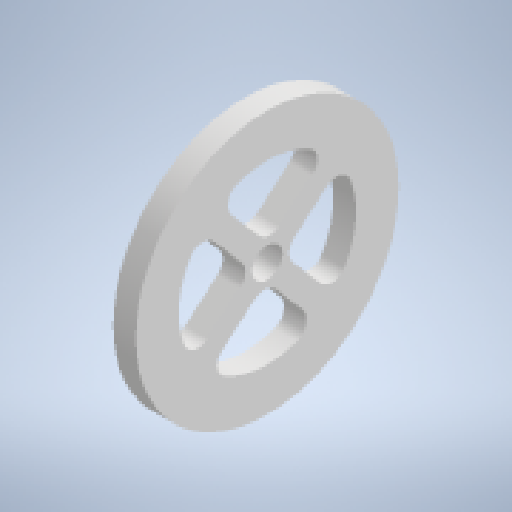
# Autodesk Inventor part: Wheel
Saved by Autodesk Inventor 2025.2 (Build 292293000, 293)
## iProperties
Created: 2025-02-03
Part Number: Wheel
Material: Generic
Document SubType Name: Modeling
Designer: andre
Density: 1 g/cm^3
Appearance: Default
Author: andre
Autodesk Inventor part; units mm, degrees
ref_plane "YZ Plane" through (0, 0, 0) normal (1, 0, 0) x (0, 1, 0)
ref_plane "XZ Plane" through (0, 0, 0) normal (0, 1, 0) x (-1, 0, 0)
ref_plane "XY Plane" through (0, 0, 0) normal (0, 0, 1) x (1, 0, 0)
sketch "Sketch1" plane through (0, 0, 0) normal (1, 0, 0) x (0, 1, 0)
  arc A0 (-4.9982, 77.0065) -> (-5.7361, 67.4907) centre (5.338, 71.4184) ccw
  arc A1 (-1.7195, 77.356) -> (-4.9982, 77.0065) centre (-3.2388, 76.0553) ccw
  line L0 (-1.7195, 77.356) -> (1.9224, 73.1018)
  arc A2 (1.7037, 70.2818) -> (1.9224, 73.1018) centre (0.4031, 71.8011) ccw
  line L1 (1.7037, 70.2818) -> (-2.5505, 66.6399)
  arc A3 (-5.7361, 67.4907) -> (-2.5505, 66.6399) centre (-3.8511, 68.1592) ccw
  arc A4 (-0.2501, 61.0823) -> (9.2657, 60.3443) centre (5.338, 71.4184) ccw
  arc A5 (-0.5995, 64.3609) -> (-0.2501, 61.0823) centre (0.7011, 62.8416) ccw
  line L2 (-0.5995, 64.3609) -> (3.6547, 68.0028)
  arc A6 (6.4746, 67.7841) -> (3.6547, 68.0028) centre (4.9553, 66.4835) ccw
  line L3 (6.4746, 67.7841) -> (10.1165, 63.5299)
  arc A7 (9.2657, 60.3443) -> (10.1165, 63.5299) centre (8.5972, 62.2293) ccw
  arc A8 (15.6742, 65.8304) -> (16.4121, 75.3462) centre (5.338, 71.4184) ccw
  arc A9 (12.3955, 65.4809) -> (15.6742, 65.8304) centre (13.9148, 66.7815) ccw
  line L4 (12.3955, 65.4809) -> (8.7536, 69.7351)
  arc A10 (8.9723, 72.5551) -> (8.7536, 69.7351) centre (10.2729, 71.0357) ccw
  line L5 (8.9723, 72.5551) -> (13.2265, 76.1969)
  arc A11 (16.4121, 75.3462) -> (13.2265, 76.1969) centre (14.5271, 74.6776) ccw
  line L6 (4.2014, 75.0527) -> (0.5595, 79.3069)
  arc A12 (1.4103, 82.4925) -> (0.5595, 79.3069) centre (2.0788, 80.6076) ccw
  arc A13 (10.926, 81.7546) -> (1.4103, 82.4925) centre (5.338, 71.4184) ccw
  arc A14 (11.2755, 78.4759) -> (10.926, 81.7546) centre (9.9749, 79.9952) ccw
  line L7 (11.2755, 78.4759) -> (7.0213, 74.834)
  arc A15 (4.2014, 75.0527) -> (7.0213, 74.834) centre (5.7207, 76.3534) ccw
  circle A16 centre (5.338, 71.4184) radius 17.5001
  circle A17 centre (5.338, 71.4184) radius 2
  point P0 (0, 0)
  dimension "d2" = 4
  constraints: 32 point on circle, 18 centre point, 16 end point
  measures "d2" diameter of A17
extrude "Extrusion1" add sketch "Sketch1" along normal blind 3
body "Solid1"
